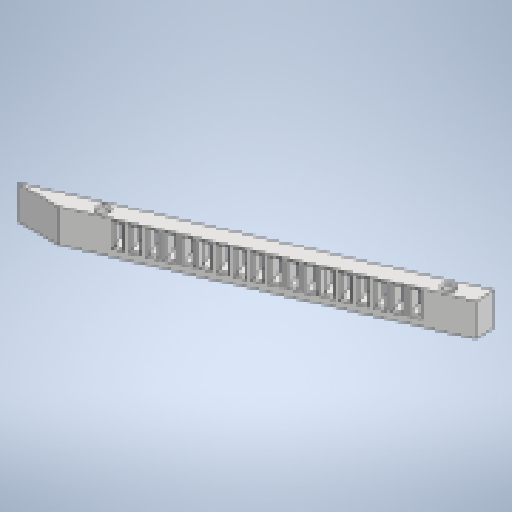
# Autodesk Inventor part: PanelRight
Saved by Autodesk Inventor 2025.2 (Build 292293000, 293)
## iProperties
Created: 2025-08-11
Part Number: PanelRight
Material: Generic
Document SubType Name: Modeling
Designer: hofma
Density: 1 g/cm^3
Appearance: Default
Author: hofma
Autodesk Inventor part; units mm, degrees
ref_plane "YZ Plane" through (0, 0, 0) normal (1, 0, 0) x (0, 1, 0)
ref_plane "XZ Plane" through (0, 0, 0) normal (0, 1, 0) x (-1, 0, 0)
ref_plane "XY Plane" through (0, 0, 0) normal (0, 0, 1) x (1, 0, 0)
sketch "Sketch1" plane through (0, 0, 0) normal (0, 1, 0) x (-1, 0, 0)
  line L0 (0, 0) -> (200, 0)
  line L1 (200, 0) -> (0, -87.5)
  line L2 (0, -87.5) -> (0, 0)
  line L3 (175.0511, 0) -> (0, -76.5848)
  dimension "d0" = 87.5
  dimension "d1" = 200
  dimension "d2" = 10
  constraints: 8 end point, 2 point on line, 1 horizontal, 1 parallel, 1 perpendicular
  measures "d0" distance of L1.end L0.start
  measures "d1" distance of L0.start L0.end
  measures "d2" distance between parallel lines of L1 L3
extrude "Extrusion1" add sketch "Sketch1" along normal mid plane 20 contours L0 L1 L2 L3
sketch "Sketch2" plane through (0, 10, 0) normal (0, 1, 0) x (1, 0, 0)
  line L0 (0, 76.5848) -> (0, 87.5) projected
  line L1 (0, 82.0424) -> (-187.5255, 0) construction
  line L2 (-200, 0) -> (-175.0511, 0) projected
  point P0 (0, 0)
  point P1 (-15, 75.4799)
  point P2 (-160, 12.0424)
  dimension "d5" = 15
  dimension "d6" = 160
  constraints: 2 end point, 2 midpoint, 2 point on line
  measures "d5" distance from line of point (-15, 75.48) L0
  measures "d6" distance from line of point (-160, 12.042) L0
hole "Hole1" at (-15, 10, -75.4799) at (-160, 10, -12.0424) direction (0, -1, 0) diameter 5.6 end through all
sketch "Sketch5" plane through (0, -10, -87.5) normal (-0.4008188, 0, -0.9161573) x (-0.9161573, 0, 0.4008188)
  line L0 (30, 18) -> (34, 18)
  line L1 (34, 18) -> (34, 5)
  line L2 (34, 5) -> (30, 5)
  line L3 (30, 5) -> (30, 18)
  line L4 (0, 0) -> (0, 20) projected
  line L5 (0, 20) -> (218.3031, 20) projected
  line L6 (218.3031, 0) -> (0, 0) projected
  point P0 (35.0716, 10)
  point P1 (0, 10)
  point P2 (30.1667, 20)
  dimension "d22" = 30
  dimension "d23" = 2
  dimension "d24" = 5
  dimension "d25" = 4
  constraints: 8 end point, 2 parallel, 1 horizontal, 1 midpoint, 1 perpendicular
  measures "d22" distance from line of L3 point (0, 10)
  measures "d23" distance between parallel lines of L5 L0
  measures "d24" distance between parallel lines of L6 L2
  measures "d25" distance between parallel lines of L1 L3
extrude "Extrusion3" cut sketch "Sketch5" against normal through all
chamfer "Chamfer1" distance 1 angle 45 8 edges at (-29.317, 8, -74.6738) (-27.4847, 1.5, -75.4754) (-29.317, -5, -74.6738) (-31.1493, 1.5, -73.8722) (-23.4765, 1.5, -66.3139) (-25.3088, -5, -65.5122) (-27.1412, 1.5, -64.7106) (-25.3088, 8, -65.5122)
pattern_linear "Rectangular Pattern1" count 18 spacing 8 along (-0.9161573, 0, 0.4008188) of "Extrusion3", "Chamfer1"
chamfer "Chamfer2" distance 1 angle 45 4 edges at (-160, 10, -14.8424) (-15, 10, -78.2799) (-160, -10, -14.8424) (-15, -10, -78.2799)
chamfer "Chamfer3" distance 1 angle 45 1 edges at (-200, 0, 0)
body "Solid1"
